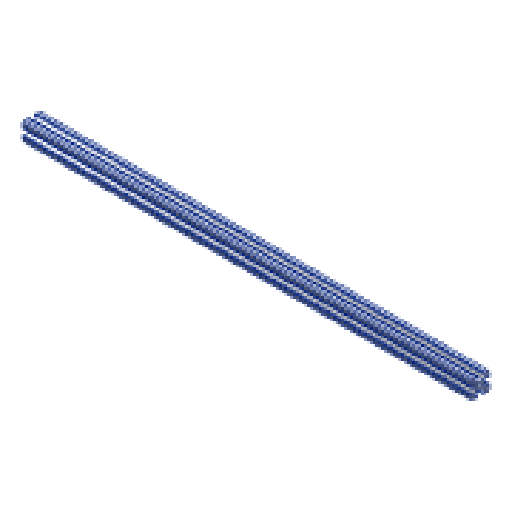
# Autodesk Inventor part: trackBase
Saved by Autodesk Inventor 2025 (Build 290162000, 162)
## iProperties
Created: 2024-07-10
Part Number: trackBase
Material: Aluminum 6061
Document SubType Name: Modeling
Designer: derm
Density: 2.7 g/cm^3
Appearance: Aluminum - Flat
Author: derm
Autodesk Inventor part; units mm, degrees
ref_plane "YZ Plane" through (0, 0, 0) normal (1, 0, 0) x (0, 1, 0)
ref_plane "XZ Plane" through (0, 0, 0) normal (0, 1, 0) x (-1, 0, 0)
ref_plane "XY Plane" through (0, 0, 0) normal (0, 0, 1) x (1, 0, 0)
sketch "Sketch1" plane through (0, 0, 0) normal (1, 0, 0) x (0, 1, 0)
  arc A0 (12.7, -5.2436) -> (12.7, -6.3485) centre (12.7, -5.796) ccw
  line L0 (12.7, -5.2436) -> (12.7, -4.1904)
  arc A1 (12.7, -4.1904) -> (11.7608, -3.2512) centre (11.7608, -4.1904) ccw
  line L1 (11.7608, -3.2512) -> (11.4294, -3.2512)
  arc A2 (11.4294, -3.2512) -> (10.4902, -4.1904) centre (11.4294, -4.1904) ccw
  line L2 (10.4902, -4.1904) -> (10.4902, -6.3485)
  arc A3 (8.6665, -7.1039) -> (10.4902, -6.3485) centre (9.4219, -6.3485) ccw
  line L3 (8.6665, -7.1039) -> (5.2999, -3.7373)
  arc A4 (4.6482, -2.164) -> (5.2999, -3.7373) centre (6.8732, -2.164) ccw
  line L4 (4.6482, -2.164) -> (4.6482, 2.164)
  arc A5 (5.2999, 3.7373) -> (4.6482, 2.164) centre (6.8732, 2.164) ccw
  line L5 (8.6665, 7.1039) -> (5.2999, 3.7373)
  arc A6 (10.4902, 6.3485) -> (8.6665, 7.1039) centre (9.4219, 6.3485) ccw
  line L6 (10.4902, 4.1904) -> (10.4902, 6.3485)
  arc A7 (10.4902, 4.1904) -> (11.4294, 3.2512) centre (11.4294, 4.1904) ccw
  line L7 (11.7608, 3.2512) -> (11.4294, 3.2512)
  arc A8 (11.7608, 3.2512) -> (12.7, 4.1904) centre (11.7608, 4.1904) ccw
  line L8 (12.7, 5.2436) -> (12.7, 4.1904)
  arc A9 (12.7, 6.3485) -> (12.7, 5.2436) centre (12.7, 5.796) ccw
  line L9 (12.7, 9.8037) -> (12.7, 6.3485)
  arc A10 (12.58, 10.8954) -> (12.7, 9.8037) centre (12.7, 10.3562) ccw
  arc A11 (12.58, 10.8954) -> (10.8954, 12.58) centre (10.1173, 10.1173) ccw
  arc A12 (9.8037, 12.7) -> (10.8954, 12.58) centre (10.3562, 12.7) ccw
  line L10 (6.3485, 12.7) -> (9.8037, 12.7)
  arc A13 (5.2436, 12.7) -> (6.3485, 12.7) centre (5.796, 12.7) ccw
  line L11 (4.1904, 12.7) -> (5.2436, 12.7)
  arc A14 (4.1904, 12.7) -> (3.2512, 11.7608) centre (4.1904, 11.7608) ccw
  line L12 (3.2512, 11.4294) -> (3.2512, 11.7608)
  arc A15 (3.2512, 11.4294) -> (4.1904, 10.4902) centre (4.1904, 11.4294) ccw
  line L13 (6.3485, 10.4902) -> (4.1904, 10.4902)
  arc A16 (7.1039, 8.6665) -> (6.3485, 10.4902) centre (6.3485, 9.4219) ccw
  line L14 (3.7373, 5.2999) -> (7.1039, 8.6665)
  arc A17 (2.164, 4.6482) -> (3.7373, 5.2999) centre (2.164, 6.8732) ccw
  line L15 (-2.164, 4.6482) -> (2.164, 4.6482)
  arc A18 (-3.7373, 5.2999) -> (-2.164, 4.6482) centre (-2.164, 6.8732) ccw
  line L16 (-3.7373, 5.2999) -> (-7.1039, 8.6665)
  arc A19 (-6.3485, 10.4902) -> (-7.1039, 8.6665) centre (-6.3485, 9.4219) ccw
  line L17 (-6.3485, 10.4902) -> (-4.1904, 10.4902)
  arc A20 (-4.1904, 10.4902) -> (-3.2512, 11.4294) centre (-4.1904, 11.4294) ccw
  line L18 (-3.2512, 11.4294) -> (-3.2512, 11.7608)
  arc A21 (-3.2512, 11.7608) -> (-4.1904, 12.7) centre (-4.1904, 11.7608) ccw
  line L19 (-4.1904, 12.7) -> (-5.2436, 12.7)
  arc A22 (-6.3485, 12.7) -> (-5.2436, 12.7) centre (-5.796, 12.7) ccw
  line L20 (-6.3485, 12.7) -> (-9.8037, 12.7)
  arc A23 (-10.8954, 12.58) -> (-9.8037, 12.7) centre (-10.3562, 12.7) ccw
  arc A24 (-10.8954, 12.58) -> (-12.58, 10.8954) centre (-10.1173, 10.1173) ccw
  arc A25 (-12.7, 9.8037) -> (-12.58, 10.8954) centre (-12.7, 10.3562) ccw
  line L21 (-12.7, 9.8037) -> (-12.7, 6.3485)
  arc A26 (-12.7, 5.2436) -> (-12.7, 6.3485) centre (-12.7, 5.796) ccw
  line L22 (-12.7, 5.2436) -> (-12.7, 4.1904)
  arc A27 (-12.7, 4.1904) -> (-11.7608, 3.2512) centre (-11.7608, 4.1904) ccw
  line L23 (-11.7608, 3.2512) -> (-11.4294, 3.2512)
  arc A28 (-11.4294, 3.2512) -> (-10.4902, 4.1904) centre (-11.4294, 4.1904) ccw
  line L24 (-10.4902, 4.1904) -> (-10.4902, 6.3485)
  arc A29 (-8.6665, 7.1039) -> (-10.4902, 6.3485) centre (-9.4219, 6.3485) ccw
  line L25 (-8.6665, 7.1039) -> (-5.2999, 3.7373)
  arc A30 (-4.6482, 2.164) -> (-5.2999, 3.7373) centre (-6.8732, 2.164) ccw
  line L26 (-4.6482, -2.164) -> (-4.6482, 2.164)
  arc A31 (-5.2999, -3.7373) -> (-4.6482, -2.164) centre (-6.8732, -2.164) ccw
  line L27 (-8.6665, -7.1039) -> (-5.2999, -3.7373)
  arc A32 (-10.4902, -6.3485) -> (-8.6665, -7.1039) centre (-9.4219, -6.3485) ccw
  line L28 (-10.4902, -4.1904) -> (-10.4902, -6.3485)
  arc A33 (-10.4902, -4.1904) -> (-11.4294, -3.2512) centre (-11.4294, -4.1904) ccw
  line L29 (-11.7608, -3.2512) -> (-11.4294, -3.2512)
  arc A34 (-11.7608, -3.2512) -> (-12.7, -4.1904) centre (-11.7608, -4.1904) ccw
  line L30 (-12.7, -5.2436) -> (-12.7, -4.1904)
  arc A35 (-12.7, -6.3485) -> (-12.7, -5.2436) centre (-12.7, -5.796) ccw
  line L31 (-12.7, -9.8037) -> (-12.7, -6.3485)
  arc A36 (-12.58, -10.8954) -> (-12.7, -9.8037) centre (-12.7, -10.3562) ccw
  arc A37 (-12.58, -10.8954) -> (-10.8954, -12.58) centre (-10.1173, -10.1173) ccw
  arc A38 (-9.8037, -12.7) -> (-10.8954, -12.58) centre (-10.3562, -12.7) ccw
  line L32 (-6.3485, -12.7) -> (-9.8037, -12.7)
  arc A39 (-5.2436, -12.7) -> (-6.3485, -12.7) centre (-5.796, -12.7) ccw
  line L33 (-4.1904, -12.7) -> (-5.2436, -12.7)
  arc A40 (-4.1904, -12.7) -> (-3.2512, -11.7608) centre (-4.1904, -11.7608) ccw
  line L34 (-3.2512, -11.4294) -> (-3.2512, -11.7608)
  arc A41 (-3.2512, -11.4294) -> (-4.1904, -10.4902) centre (-4.1904, -11.4294) ccw
  line L35 (-6.3485, -10.4902) -> (-4.1904, -10.4902)
  arc A42 (-7.1039, -8.6665) -> (-6.3485, -10.4902) centre (-6.3485, -9.4219) ccw
  line L36 (-3.7373, -5.2999) -> (-7.1039, -8.6665)
  arc A43 (-2.164, -4.6482) -> (-3.7373, -5.2999) centre (-2.164, -6.8732) ccw
  line L37 (-2.164, -4.6482) -> (2.164, -4.6482)
  arc A44 (3.7373, -5.2999) -> (2.164, -4.6482) centre (2.164, -6.8732) ccw
  line L38 (3.7373, -5.2999) -> (7.1039, -8.6665)
  arc A45 (6.3485, -10.4902) -> (7.1039, -8.6665) centre (6.3485, -9.4219) ccw
  line L39 (6.3485, -10.4902) -> (4.1904, -10.4902)
  arc A46 (4.1904, -10.4902) -> (3.2512, -11.4294) centre (4.1904, -11.4294) ccw
  line L40 (3.2512, -11.4294) -> (3.2512, -11.7608)
  arc A47 (3.2512, -11.7608) -> (4.1904, -12.7) centre (4.1904, -11.7608) ccw
  line L41 (4.1904, -12.7) -> (5.2436, -12.7)
  arc A48 (6.3485, -12.7) -> (5.2436, -12.7) centre (5.796, -12.7) ccw
  line L42 (6.3485, -12.7) -> (9.8037, -12.7)
  arc A49 (10.8954, -12.58) -> (9.8037, -12.7) centre (10.3562, -12.7) ccw
  arc A50 (10.8954, -12.58) -> (12.58, -10.8954) centre (10.1173, -10.1173) ccw
  arc A51 (12.7, -9.8037) -> (12.58, -10.8954) centre (12.7, -10.3562) ccw
  line L43 (12.7, -9.8037) -> (12.7, -6.3485)
  circle A52 centre (0, 0) radius 2.6035
  point P0 (0, 0)
  point P1 (0, 0)
  constraints: 104 point on circle, 88 end point, 53 centre point
extrude "Extrusion1" add sketch "Sketch1" against normal blind 609.6
body "Solid1"
